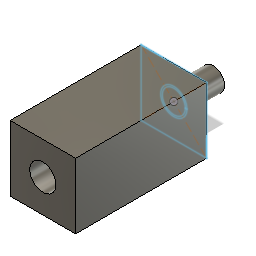
Board support post v2 (Autodesk Fusion 360 design; units mm, degrees)
Autodesk Fusion 360 part; units mm, degrees
sketch "Sketch1" plane through (0, 0, 0) normal (0, 0, 1) x (1, 0, 0)
  circle A0 centre (0, 0) radius 1.016
  circle A1 centre (0, 0) radius 0.889
  line L0 (2.54, 2.54) -> (-2.54, 2.54)
  line L1 (-2.54, 2.54) -> (-2.54, -2.54)
  line L2 (-2.54, -2.54) -> (2.54, -2.54)
  line L3 (2.54, -2.54) -> (2.54, 2.54)
  line L4 (2.54, 2.54) -> (-2.54, -2.54) construction
  line L5 (-2.54, 2.54) -> (2.54, -2.54) construction
  dimension "d2" = 2.032
  dimension "d7" = 1.778
  dimension "d10" = 5.08
  dimension "d11" = 5.08
  constraint perpendicular L0 L1
  constraint parallel L0 L2
  constraint parallel L1 L3
  constraint horizontal L0
  constraint coincident L4 A0.centre
  constraint coincident L5 A0.centre
  measures "d2" diameter of A0
  measures "d7" diameter of A1
  measures "d10" distance of L1.end L2.end
  measures "d11" distance of L0.end L1.end
extrude "Extrude1" add sketch "Sketch1" along normal blind 10.16 contours L0 L1 L2 L3
extrude "Extrude2" add sketch "Sketch1" along normal blind 4.572 contours A0 | A1
extrude "Extrude3" add sketch "Sketch1" against normal blind 3.048 contours A1
